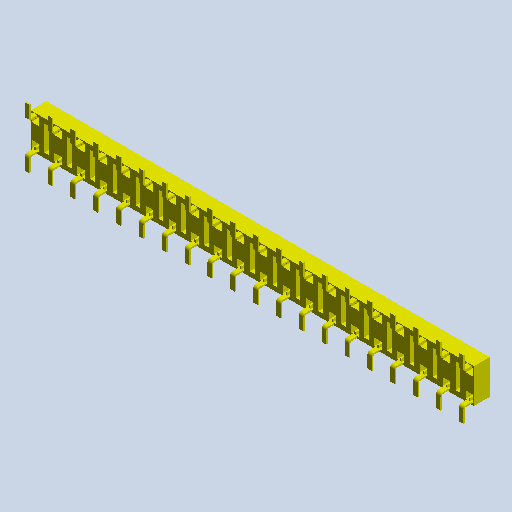
# Autodesk Inventor part: C-132-12-20-DV
Saved by Autodesk Inventor 2022 (Build 260153000, 153)
## iProperties
Category: PARTsolutions
Company: SAMTEC
Part Number: C-132-12-20-DV
Material: Generic
Catalog Web Link: www.cadenas.de
Description: C-132-Pins
Vendor: SAMTEC
Document SubType Name: Modeling
Designer: partserver
Manufacturer: SAMTEC
Mass: 0.2484 g
Surface Area: 10.7462 cm^2
Volume: 0.2484 cm^3
Density: 1 g/cm^3
Appearance: PSOLRGB-255-255-0
PSOL_IDENT_0: {$CADENAS_DATA\23d-libs\samtec\modelling\hle\parts\hle_pins.prj},176 {VTYP=3D},{NB=C-132-12-20-DV},{
PSOL_IDENT_1: LINA=C-132-12-20-DV},{NN=C-132},{DATE=08.04.2016 05:41:50},{GEOMDATE=08.04.2016 05:31:00},{VERSION=}
PSOL_IDENT_2: ,{LINEID=10},{WBVAR=POS,ESOPT},{WBNUMERIC=}  {NB=C-132-12-20-DV},{LINA=C-132-12-20-DV},{KT=DUMMY},{P
PSOL_IDENT_3: N=C-132-12-20-DV},{SERIES=HLE},{POSALG=  '02' , '-02' , '03' , '-03' , '04' , '-04' , '05' , '-05' ,
PSOL_IDENT_4: '06' , '-06' , '07' , '-07' , '08' , '-08' , '09' , '-09' , '10' , '-10' , '11' , '-11' , '12' , '-
PSOL_IDENT_5: 12' , '13' , '-13' , '14' , '-14' , '15' , '-15' , '16' , '-16' , '17' , '-17' , '18' , '-18' , '19'
PSOL_IDENT_6: , '-19' , '20' , '-20' , '21' , '-21' , '22' , '-22' , '23' , '-23' , '24' , '-24' , '25' , '-25' ,
PSOL_IDENT_7: '26' , '-26' , '27' , '-27' , '28' , '-28' , '29' , '-29' , '30' , '-30' , '31' , '-31' , '32' , '-
PSOL_IDENT_8: 32' , '33' , '-33' , '34' , '-34' , '35' , '-35' , '36' , '-36' , '37' , '-37' , '38' , '-38' , '39'
PSOL_IDENT_9: , '-39' , '40' , '-40'  , '41' , '-41' , '42' , '-42' , '43' , '-43' , '44' , '-44' , '45' , '-45'
PSOL_IDENT_10: , '46' , '-46' , '47' , '-47' , '48' , '-48' , '49' , '-49' , '50' , '-50'   , '51' , '-51' , '52' ,
PSOL_IDENT_11: '-52' , '53' , '-53' , '54' , '-54' , '55' , '-55' , '56' , '-56' , '57' , '-57' , '58' , '-58' , '
PSOL_IDENT_12: 59' , '-59' , '60' , '-60'  , '61' , '-61' , '62' , '-62' , '63' , '-63' , '64' , '-64' , '65' , '-6
PSOL_IDENT_13: 5' , '66' , '-66' , '67' , '-67' , '68' , '-68' , '69' , '-69' , '70' , '-70'  , '71' , '-71' , '72'
PSOL_IDENT_14: , '-72' , '73' , '-73' , '74' , '-74' , '75' , '-75'   },{POS=20},{LSALG=  '02' , '-02 - Surface Mo
PSOL_IDENT_15: unt'  },{LS=02},{ROPTALG=   'DV' , '-DV - Double Vertical'   },{ROPT=DV},{ESOPT=},{A=0.144},{B=0.138
PSOL_IDENT_16: },{L=2.000},{PINS=20},{H2=0.030},{W=0.2000},{PINH=0.025},{PINL=0.2590},{PINW=0.020},{PITCH=0.1000},{
PSOL_IDENT_17: PITCH2=0.1000},{X=0.045},{ESOPTPN=}
NB: C-132-12-20-DV
NN: C-132
NT: Pins
NBSYN: $PN.
LINA: C-132-12-20-DV
CATALOG: Samtec
PN: C-132-12-20-DV
SERIES: HLE
POS: -20
LS: 02
ROPT: DV
ESOPT: Standard
A: 0.144
B: 0.138
L: 2
H2: 0.03
W: 0.2
PINH: 0.025
PINL: 0.259
PINW: 0.02
PITCH: 0.1
PITCH2: 0.1
X: 0.045
SUPPLIER: SAMTEC
ARTICLENO: C-132-12-20-DV
BOMINFO: C-132-12-20-DV
CREATOR: CADENAS GmbH
Title: C-132-12-20-DV
Author: Cadenas PARTsolutions
Comments: Pins
Autodesk Inventor part; units mm, degrees
sketch "Sketch_11" plane through (0, 2.5146, 0) normal (0, 1, 0) x (1, 0, 0)
  line L0 (-24.638, 1.9177) -> (-24.638, -1.9177)
  line L1 (-24.638, -1.9177) -> (24.638, -1.9177)
  line L2 (24.638, -1.9177) -> (24.638, 1.9177)
  line L3 (24.638, 1.9177) -> (-24.638, 1.9177)
  line L4 (23.7236, -0.8636) -> (23.7236, -1.6764)
  line L5 (23.7236, -1.6764) -> (24.0538, -1.6764)
  line L6 (24.0538, -1.6764) -> (24.0538, -1.3716)
  line L7 (24.0538, -1.3716) -> (24.2062, -1.3716)
  line L8 (24.2062, -1.3716) -> (24.2062, -1.6764)
  line L9 (24.2062, -1.6764) -> (24.5364, -1.6764)
  line L10 (24.5364, -1.6764) -> (24.5364, -0.8636)
  line L11 (24.5364, -0.8636) -> (23.7236, -0.8636)
  line L12 (23.7236, 0.8636) -> (24.5364, 0.8636)
  line L13 (24.5364, 0.8636) -> (24.5364, 1.6764)
  line L14 (24.5364, 1.6764) -> (24.2062, 1.6764)
  line L15 (24.2062, 1.6764) -> (24.2062, 1.3716)
  line L16 (24.2062, 1.3716) -> (24.0538, 1.3716)
  line L17 (24.0538, 1.3716) -> (24.0538, 1.6764)
  line L18 (24.0538, 1.6764) -> (23.7236, 1.6764)
  line L19 (23.7236, 1.6764) -> (23.7236, 0.8636)
  line L20 (22.606, 1.397) -> (22.606, -1.397)
  line L21 (22.606, -1.397) -> (23.114, -1.397)
  line L22 (23.114, -1.397) -> (23.114, 1.397)
  line L23 (23.114, 1.397) -> (22.606, 1.397)
  line L24 (21.1836, -0.8636) -> (21.1836, -1.6764)
  line L25 (21.1836, -1.6764) -> (21.5138, -1.6764)
  line L26 (21.5138, -1.6764) -> (21.5138, -1.3716)
  line L27 (21.5138, -1.3716) -> (21.6662, -1.3716)
  line L28 (21.6662, -1.3716) -> (21.6662, -1.6764)
  line L29 (21.6662, -1.6764) -> (21.9964, -1.6764)
  line L30 (21.9964, -1.6764) -> (21.9964, -0.8636)
  line L31 (21.9964, -0.8636) -> (21.1836, -0.8636)
  line L32 (21.1836, 0.8636) -> (21.9964, 0.8636)
  line L33 (21.9964, 0.8636) -> (21.9964, 1.6764)
  line L34 (21.9964, 1.6764) -> (21.6662, 1.6764)
  line L35 (21.6662, 1.6764) -> (21.6662, 1.3716)
  line L36 (21.6662, 1.3716) -> (21.5138, 1.3716)
  line L37 (21.5138, 1.3716) -> (21.5138, 1.6764)
  line L38 (21.5138, 1.6764) -> (21.1836, 1.6764)
  line L39 (21.1836, 1.6764) -> (21.1836, 0.8636)
  line L40 (20.066, 1.397) -> (20.066, -1.397)
  line L41 (20.066, -1.397) -> (20.574, -1.397)
  line L42 (20.574, -1.397) -> (20.574, 1.397)
  line L43 (20.574, 1.397) -> (20.066, 1.397)
  line L44 (18.6436, -0.8636) -> (18.6436, -1.6764)
  line L45 (18.6436, -1.6764) -> (18.9738, -1.6764)
  line L46 (18.9738, -1.6764) -> (18.9738, -1.3716)
  line L47 (18.9738, -1.3716) -> (19.1262, -1.3716)
  line L48 (19.1262, -1.3716) -> (19.1262, -1.6764)
  line L49 (19.1262, -1.6764) -> (19.4564, -1.6764)
  line L50 (19.4564, -1.6764) -> (19.4564, -0.8636)
  line L51 (19.4564, -0.8636) -> (18.6436, -0.8636)
  line L52 (18.6436, 0.8636) -> (19.4564, 0.8636)
  line L53 (19.4564, 0.8636) -> (19.4564, 1.6764)
  line L54 (19.4564, 1.6764) -> (19.1262, 1.6764)
  line L55 (19.1262, 1.6764) -> (19.1262, 1.3716)
  line L56 (19.1262, 1.3716) -> (18.9738, 1.3716)
  line L57 (18.9738, 1.3716) -> (18.9738, 1.6764)
  line L58 (18.9738, 1.6764) -> (18.6436, 1.6764)
  line L59 (18.6436, 1.6764) -> (18.6436, 0.8636)
  line L60 (17.526, 1.397) -> (17.526, -1.397)
  line L61 (17.526, -1.397) -> (18.034, -1.397)
  line L62 (18.034, -1.397) -> (18.034, 1.397)
  line L63 (18.034, 1.397) -> (17.526, 1.397)
  line L64 (16.1036, -0.8636) -> (16.1036, -1.6764)
  line L65 (16.1036, -1.6764) -> (16.4338, -1.6764)
  line L66 (16.4338, -1.6764) -> (16.4338, -1.3716)
  line L67 (16.4338, -1.3716) -> (16.5862, -1.3716)
  line L68 (16.5862, -1.3716) -> (16.5862, -1.6764)
  line L69 (16.5862, -1.6764) -> (16.9164, -1.6764)
  line L70 (16.9164, -1.6764) -> (16.9164, -0.8636)
  line L71 (16.9164, -0.8636) -> (16.1036, -0.8636)
  line L72 (16.1036, 0.8636) -> (16.9164, 0.8636)
  line L73 (16.9164, 0.8636) -> (16.9164, 1.6764)
  line L74 (16.9164, 1.6764) -> (16.5862, 1.6764)
  line L75 (16.5862, 1.6764) -> (16.5862, 1.3716)
  line L76 (16.5862, 1.3716) -> (16.4338, 1.3716)
  line L77 (16.4338, 1.3716) -> (16.4338, 1.6764)
  line L78 (16.4338, 1.6764) -> (16.1036, 1.6764)
  line L79 (16.1036, 1.6764) -> (16.1036, 0.8636)
  line L80 (14.986, 1.397) -> (14.986, -1.397)
  line L81 (14.986, -1.397) -> (15.494, -1.397)
  line L82 (15.494, -1.397) -> (15.494, 1.397)
  line L83 (15.494, 1.397) -> (14.986, 1.397)
  line L84 (13.5636, -0.8636) -> (13.5636, -1.6764)
  line L85 (13.5636, -1.6764) -> (13.8938, -1.6764)
  line L86 (13.8938, -1.6764) -> (13.8938, -1.3716)
  line L87 (13.8938, -1.3716) -> (14.0462, -1.3716)
  line L88 (14.0462, -1.3716) -> (14.0462, -1.6764)
  line L89 (14.0462, -1.6764) -> (14.3764, -1.6764)
  line L90 (14.3764, -1.6764) -> (14.3764, -0.8636)
  line L91 (14.3764, -0.8636) -> (13.5636, -0.8636)
  line L92 (13.5636, 0.8636) -> (14.3764, 0.8636)
  line L93 (14.3764, 0.8636) -> (14.3764, 1.6764)
  line L94 (14.3764, 1.6764) -> (14.0462, 1.6764)
  line L95 (14.0462, 1.6764) -> (14.0462, 1.3716)
  line L96 (14.0462, 1.3716) -> (13.8938, 1.3716)
  line L97 (13.8938, 1.3716) -> (13.8938, 1.6764)
  line L98 (13.8938, 1.6764) -> (13.5636, 1.6764)
  line L99 (13.5636, 1.6764) -> (13.5636, 0.8636)
  line L100 (12.446, 1.397) -> (12.446, -1.397)
  line L101 (12.446, -1.397) -> (12.954, -1.397)
  line L102 (12.954, -1.397) -> (12.954, 1.397)
  line L103 (12.954, 1.397) -> (12.446, 1.397)
  line L104 (11.0236, -0.8636) -> (11.0236, -1.6764)
  line L105 (11.0236, -1.6764) -> (11.3538, -1.6764)
  line L106 (11.3538, -1.6764) -> (11.3538, -1.3716)
  line L107 (11.3538, -1.3716) -> (11.5062, -1.3716)
  line L108 (11.5062, -1.3716) -> (11.5062, -1.6764)
  line L109 (11.5062, -1.6764) -> (11.8364, -1.6764)
  line L110 (11.8364, -1.6764) -> (11.8364, -0.8636)
  line L111 (11.8364, -0.8636) -> (11.0236, -0.8636)
  line L112 (11.0236, 0.8636) -> (11.8364, 0.8636)
  line L113 (11.8364, 0.8636) -> (11.8364, 1.6764)
  line L114 (11.8364, 1.6764) -> (11.5062, 1.6764)
  line L115 (11.5062, 1.6764) -> (11.5062, 1.3716)
  line L116 (11.5062, 1.3716) -> (11.3538, 1.3716)
  line L117 (11.3538, 1.3716) -> (11.3538, 1.6764)
  line L118 (11.3538, 1.6764) -> (11.0236, 1.6764)
  line L119 (11.0236, 1.6764) -> (11.0236, 0.8636)
  line L120 (9.906, 1.397) -> (9.906, -1.397)
  line L121 (9.906, -1.397) -> (10.414, -1.397)
  line L122 (10.414, -1.397) -> (10.414, 1.397)
  line L123 (10.414, 1.397) -> (9.906, 1.397)
  line L124 (8.4836, -0.8636) -> (8.4836, -1.6764)
  line L125 (8.4836, -1.6764) -> (8.8138, -1.6764)
  line L126 (8.8138, -1.6764) -> (8.8138, -1.3716)
  line L127 (8.8138, -1.3716) -> (8.9662, -1.3716)
  line L128 (8.9662, -1.3716) -> (8.9662, -1.6764)
  line L129 (8.9662, -1.6764) -> (9.2964, -1.6764)
  line L130 (9.2964, -1.6764) -> (9.2964, -0.8636)
  line L131 (9.2964, -0.8636) -> (8.4836, -0.8636)
  line L132 (8.4836, 0.8636) -> (9.2964, 0.8636)
  line L133 (9.2964, 0.8636) -> (9.2964, 1.6764)
  line L134 (9.2964, 1.6764) -> (8.9662, 1.6764)
  line L135 (8.9662, 1.6764) -> (8.9662, 1.3716)
  line L136 (8.9662, 1.3716) -> (8.8138, 1.3716)
  line L137 (8.8138, 1.3716) -> (8.8138, 1.6764)
  line L138 (8.8138, 1.6764) -> (8.4836, 1.6764)
  line L139 (8.4836, 1.6764) -> (8.4836, 0.8636)
  line L140 (7.366, 1.397) -> (7.366, -1.397)
  line L141 (7.366, -1.397) -> (7.874, -1.397)
  line L142 (7.874, -1.397) -> (7.874, 1.397)
  line L143 (7.874, 1.397) -> (7.366, 1.397)
  line L144 (5.9436, -0.8636) -> (5.9436, -1.6764)
  line L145 (5.9436, -1.6764) -> (6.2738, -1.6764)
  line L146 (6.2738, -1.6764) -> (6.2738, -1.3716)
  line L147 (6.2738, -1.3716) -> (6.4262, -1.3716)
  line L148 (6.4262, -1.3716) -> (6.4262, -1.6764)
  line L149 (6.4262, -1.6764) -> (6.7564, -1.6764)
  line L150 (6.7564, -1.6764) -> (6.7564, -0.8636)
  line L151 (6.7564, -0.8636) -> (5.9436, -0.8636)
  line L152 (5.9436, 0.8636) -> (6.7564, 0.8636)
  line L153 (6.7564, 0.8636) -> (6.7564, 1.6764)
  line L154 (6.7564, 1.6764) -> (6.4262, 1.6764)
  line L155 (6.4262, 1.6764) -> (6.4262, 1.3716)
  line L156 (6.4262, 1.3716) -> (6.2738, 1.3716)
  line L157 (6.2738, 1.3716) -> (6.2738, 1.6764)
  line L158 (6.2738, 1.6764) -> (5.9436, 1.6764)
  line L159 (5.9436, 1.6764) -> (5.9436, 0.8636)
  line L160 (4.826, 1.397) -> (4.826, -1.397)
  line L161 (4.826, -1.397) -> (5.334, -1.397)
  line L162 (5.334, -1.397) -> (5.334, 1.397)
  line L163 (5.334, 1.397) -> (4.826, 1.397)
  line L164 (3.4036, -0.8636) -> (3.4036, -1.6764)
  line L165 (3.4036, -1.6764) -> (3.7338, -1.6764)
  line L166 (3.7338, -1.6764) -> (3.7338, -1.3716)
  line L167 (3.7338, -1.3716) -> (3.8862, -1.3716)
  line L168 (3.8862, -1.3716) -> (3.8862, -1.6764)
  line L169 (3.8862, -1.6764) -> (4.2164, -1.6764)
  line L170 (4.2164, -1.6764) -> (4.2164, -0.8636)
  line L171 (4.2164, -0.8636) -> (3.4036, -0.8636)
  line L172 (3.4036, 0.8636) -> (4.2164, 0.8636)
  line L173 (4.2164, 0.8636) -> (4.2164, 1.6764)
  line L174 (4.2164, 1.6764) -> (3.8862, 1.6764)
  line L175 (3.8862, 1.6764) -> (3.8862, 1.3716)
  line L176 (3.8862, 1.3716) -> (3.7338, 1.3716)
  line L177 (3.7338, 1.3716) -> (3.7338, 1.6764)
  line L178 (3.7338, 1.6764) -> (3.4036, 1.6764)
  line L179 (3.4036, 1.6764) -> (3.4036, 0.8636)
  line L180 (2.286, 1.397) -> (2.286, -1.397)
  line L181 (2.286, -1.397) -> (2.794, -1.397)
  line L182 (2.794, -1.397) -> (2.794, 1.397)
  line L183 (2.794, 1.397) -> (2.286, 1.397)
  line L184 (0.8636, -0.8636) -> (0.8636, -1.6764)
  line L185 (0.8636, -1.6764) -> (1.1938, -1.6764)
  line L186 (1.1938, -1.6764) -> (1.1938, -1.3716)
  line L187 (1.1938, -1.3716) -> (1.3462, -1.3716)
  line L188 (1.3462, -1.3716) -> (1.3462, -1.6764)
  line L189 (1.3462, -1.6764) -> (1.6764, -1.6764)
  line L190 (1.6764, -1.6764) -> (1.6764, -0.8636)
  line L191 (1.6764, -0.8636) -> (0.8636, -0.8636)
  line L192 (0.8636, 0.8636) -> (1.6764, 0.8636)
  line L193 (1.6764, 0.8636) -> (1.6764, 1.6764)
  line L194 (1.6764, 1.6764) -> (1.3462, 1.6764)
  line L195 (1.3462, 1.6764) -> (1.3462, 1.3716)
  line L196 (1.3462, 1.3716) -> (1.1938, 1.3716)
  line L197 (1.1938, 1.3716) -> (1.1938, 1.6764)
  line L198 (1.1938, 1.6764) -> (0.8636, 1.6764)
  line L199 (0.8636, 1.6764) -> (0.8636, 0.8636)
  line L200 (-0.254, 1.397) -> (-0.254, -1.397)
  line L201 (-0.254, -1.397) -> (0.254, -1.397)
  line L202 (0.254, -1.397) -> (0.254, 1.397)
  line L203 (0.254, 1.397) -> (-0.254, 1.397)
  line L204 (-1.6764, -0.8636) -> (-1.6764, -1.6764)
  line L205 (-1.6764, -1.6764) -> (-1.3462, -1.6764)
  line L206 (-1.3462, -1.6764) -> (-1.3462, -1.3716)
  line L207 (-1.3462, -1.3716) -> (-1.1938, -1.3716)
  line L208 (-1.1938, -1.3716) -> (-1.1938, -1.6764)
  line L209 (-1.1938, -1.6764) -> (-0.8636, -1.6764)
  line L210 (-0.8636, -1.6764) -> (-0.8636, -0.8636)
  line L211 (-0.8636, -0.8636) -> (-1.6764, -0.8636)
  line L212 (-1.6764, 0.8636) -> (-0.8636, 0.8636)
  line L213 (-0.8636, 0.8636) -> (-0.8636, 1.6764)
  line L214 (-0.8636, 1.6764) -> (-1.1938, 1.6764)
  line L215 (-1.1938, 1.6764) -> (-1.1938, 1.3716)
  line L216 (-1.1938, 1.3716) -> (-1.3462, 1.3716)
  line L217 (-1.3462, 1.3716) -> (-1.3462, 1.6764)
  line L218 (-1.3462, 1.6764) -> (-1.6764, 1.6764)
  line L219 (-1.6764, 1.6764) -> (-1.6764, 0.8636)
  line L220 (-2.794, 1.397) -> (-2.794, -1.397)
  line L221 (-2.794, -1.397) -> (-2.286, -1.397)
  line L222 (-2.286, -1.397) -> (-2.286, 1.397)
  line L223 (-2.286, 1.397) -> (-2.794, 1.397)
  line L224 (-4.2164, -0.8636) -> (-4.2164, -1.6764)
  line L225 (-4.2164, -1.6764) -> (-3.8862, -1.6764)
  line L226 (-3.8862, -1.6764) -> (-3.8862, -1.3716)
  line L227 (-3.8862, -1.3716) -> (-3.7338, -1.3716)
  line L228 (-3.7338, -1.3716) -> (-3.7338, -1.6764)
  line L229 (-3.7338, -1.6764) -> (-3.4036, -1.6764)
  line L230 (-3.4036, -1.6764) -> (-3.4036, -0.8636)
  line L231 (-3.4036, -0.8636) -> (-4.2164, -0.8636)
  line L232 (-4.2164, 0.8636) -> (-3.4036, 0.8636)
  line L233 (-3.4036, 0.8636) -> (-3.4036, 1.6764)
  line L234 (-3.4036, 1.6764) -> (-3.7338, 1.6764)
  line L235 (-3.7338, 1.6764) -> (-3.7338, 1.3716)
  line L236 (-3.7338, 1.3716) -> (-3.8862, 1.3716)
  line L237 (-3.8862, 1.3716) -> (-3.8862, 1.6764)
  line L238 (-3.8862, 1.6764) -> (-4.2164, 1.6764)
  line L239 (-4.2164, 1.6764) -> (-4.2164, 0.8636)
  line L240 (-5.334, 1.397) -> (-5.334, -1.397)
  line L241 (-5.334, -1.397) -> (-4.826, -1.397)
  line L242 (-4.826, -1.397) -> (-4.826, 1.397)
  line L243 (-4.826, 1.397) -> (-5.334, 1.397)
  line L244 (-6.7564, -0.8636) -> (-6.7564, -1.6764)
  line L245 (-6.7564, -1.6764) -> (-6.4262, -1.6764)
  line L246 (-6.4262, -1.6764) -> (-6.4262, -1.3716)
  line L247 (-6.4262, -1.3716) -> (-6.2738, -1.3716)
  line L248 (-6.2738, -1.3716) -> (-6.2738, -1.6764)
  line L249 (-6.2738, -1.6764) -> (-5.9436, -1.6764)
  line L250 (-5.9436, -1.6764) -> (-5.9436, -0.8636)
  line L251 (-5.9436, -0.8636) -> (-6.7564, -0.8636)
  line L252 (-6.7564, 0.8636) -> (-5.9436, 0.8636)
  line L253 (-5.9436, 0.8636) -> (-5.9436, 1.6764)
  line L254 (-5.9436, 1.6764) -> (-6.2738, 1.6764)
  line L255 (-6.2738, 1.6764) -> (-6.2738, 1.3716)
  line L256 (-6.2738, 1.3716) -> (-6.4262, 1.3716)
  line L257 (-6.4262, 1.3716) -> (-6.4262, 1.6764)
  line L258 (-6.4262, 1.6764) -> (-6.7564, 1.6764)
  line L259 (-6.7564, 1.6764) -> (-6.7564, 0.8636)
  line L260 (-7.874, 1.397) -> (-7.874, -1.397)
  line L261 (-7.874, -1.397) -> (-7.366, -1.397)
  line L262 (-7.366, -1.397) -> (-7.366, 1.397)
  line L263 (-7.366, 1.397) -> (-7.874, 1.397)
  line L264 (-9.2964, -0.8636) -> (-9.2964, -1.6764)
  line L265 (-9.2964, -1.6764) -> (-8.9662, -1.6764)
  line L266 (-8.9662, -1.6764) -> (-8.9662, -1.3716)
  line L267 (-8.9662, -1.3716) -> (-8.8138, -1.3716)
  line L268 (-8.8138, -1.3716) -> (-8.8138, -1.6764)
  line L269 (-8.8138, -1.6764) -> (-8.4836, -1.6764)
  line L270 (-8.4836, -1.6764) -> (-8.4836, -0.8636)
  line L271 (-8.4836, -0.8636) -> (-9.2964, -0.8636)
  line L272 (-9.2964, 0.8636) -> (-8.4836, 0.8636)
  line L273 (-8.4836, 0.8636) -> (-8.4836, 1.6764)
  line L274 (-8.4836, 1.6764) -> (-8.8138, 1.6764)
  line L275 (-8.8138, 1.6764) -> (-8.8138, 1.3716)
  line L276 (-8.8138, 1.3716) -> (-8.9662, 1.3716)
  line L277 (-8.9662, 1.3716) -> (-8.9662, 1.6764)
  line L278 (-8.9662, 1.6764) -> (-9.2964, 1.6764)
  line L279 (-9.2964, 1.6764) -> (-9.2964, 0.8636)
  line L280 (-10.414, 1.397) -> (-10.414, -1.397)
  line L281 (-10.414, -1.397) -> (-9.906, -1.397)
  line L282 (-9.906, -1.397) -> (-9.906, 1.397)
  line L283 (-9.906, 1.397) -> (-10.414, 1.397)
  line L284 (-11.8364, -0.8636) -> (-11.8364, -1.6764)
  line L285 (-11.8364, -1.6764) -> (-11.5062, -1.6764)
  line L286 (-11.5062, -1.6764) -> (-11.5062, -1.3716)
  line L287 (-11.5062, -1.3716) -> (-11.3538, -1.3716)
  line L288 (-11.3538, -1.3716) -> (-11.3538, -1.6764)
  line L289 (-11.3538, -1.6764) -> (-11.0236, -1.6764)
  line L290 (-11.0236, -1.6764) -> (-11.0236, -0.8636)
  line L291 (-11.0236, -0.8636) -> (-11.8364, -0.8636)
  line L292 (-11.8364, 0.8636) -> (-11.0236, 0.8636)
  line L293 (-11.0236, 0.8636) -> (-11.0236, 1.6764)
  line L294 (-11.0236, 1.6764) -> (-11.3538, 1.6764)
  line L295 (-11.3538, 1.6764) -> (-11.3538, 1.3716)
  line L296 (-11.3538, 1.3716) -> (-11.5062, 1.3716)
  line L297 (-11.5062, 1.3716) -> (-11.5062, 1.6764)
  line L298 (-11.5062, 1.6764) -> (-11.8364, 1.6764)
  line L299 (-11.8364, 1.6764) -> (-11.8364, 0.8636)
  line L300 (-12.954, 1.397) -> (-12.954, -1.397)
  line L301 (-12.954, -1.397) -> (-12.446, -1.397)
  line L302 (-12.446, -1.397) -> (-12.446, 1.397)
  line L303 (-12.446, 1.397) -> (-12.954, 1.397)
  line L304 (-14.3764, -0.8636) -> (-14.3764, -1.6764)
  line L305 (-14.3764, -1.6764) -> (-14.0462, -1.6764)
  line L306 (-14.0462, -1.6764) -> (-14.0462, -1.3716)
  line L307 (-14.0462, -1.3716) -> (-13.8938, -1.3716)
  line L308 (-13.8938, -1.3716) -> (-13.8938, -1.6764)
  line L309 (-13.8938, -1.6764) -> (-13.5636, -1.6764)
  line L310 (-13.5636, -1.6764) -> (-13.5636, -0.8636)
  line L311 (-13.5636, -0.8636) -> (-14.3764, -0.8636)
  line L312 (-14.3764, 0.8636) -> (-13.5636, 0.8636)
  line L313 (-13.5636, 0.8636) -> (-13.5636, 1.6764)
  line L314 (-13.5636, 1.6764) -> (-13.8938, 1.6764)
  line L315 (-13.8938, 1.6764) -> (-13.8938, 1.3716)
  line L316 (-13.8938, 1.3716) -> (-14.0462, 1.3716)
  line L317 (-14.0462, 1.3716) -> (-14.0462, 1.6764)
  line L318 (-14.0462, 1.6764) -> (-14.3764, 1.6764)
  line L319 (-14.3764, 1.6764) -> (-14.3764, 0.8636)
  line L320 (-15.494, 1.397) -> (-15.494, -1.397)
  line L321 (-15.494, -1.397) -> (-14.986, -1.397)
  line L322 (-14.986, -1.397) -> (-14.986, 1.397)
  line L323 (-14.986, 1.397) -> (-15.494, 1.397)
  line L324 (-16.9164, -0.8636) -> (-16.9164, -1.6764)
  line L325 (-16.9164, -1.6764) -> (-16.5862, -1.6764)
  line L326 (-16.5862, -1.6764) -> (-16.5862, -1.3716)
  line L327 (-16.5862, -1.3716) -> (-16.4338, -1.3716)
  line L328 (-16.4338, -1.3716) -> (-16.4338, -1.6764)
  line L329 (-16.4338, -1.6764) -> (-16.1036, -1.6764)
  line L330 (-16.1036, -1.6764) -> (-16.1036, -0.8636)
  line L331 (-16.1036, -0.8636) -> (-16.9164, -0.8636)
  line L332 (-16.9164, 0.8636) -> (-16.1036, 0.8636)
  line L333 (-16.1036, 0.8636) -> (-16.1036, 1.6764)
  line L334 (-16.1036, 1.6764) -> (-16.4338, 1.6764)
  line L335 (-16.4338, 1.6764) -> (-16.4338, 1.3716)
  line L336 (-16.4338, 1.3716) -> (-16.5862, 1.3716)
  line L337 (-16.5862, 1.3716) -> (-16.5862, 1.6764)
  line L338 (-16.5862, 1.6764) -> (-16.9164, 1.6764)
  line L339 (-16.9164, 1.6764) -> (-16.9164, 0.8636)
  line L340 (-18.034, 1.397) -> (-18.034, -1.397)
  line L341 (-18.034, -1.397) -> (-17.526, -1.397)
  line L342 (-17.526, -1.397) -> (-17.526, 1.397)
  line L343 (-17.526, 1.397) -> (-18.034, 1.397)
  line L344 (-19.4564, -0.8636) -> (-19.4564, -1.6764)
  line L345 (-19.4564, -1.6764) -> (-19.1262, -1.6764)
  line L346 (-19.1262, -1.6764) -> (-19.1262, -1.3716)
  line L347 (-19.1262, -1.3716) -> (-18.9738, -1.3716)
  line L348 (-18.9738, -1.3716) -> (-18.9738, -1.6764)
  line L349 (-18.9738, -1.6764) -> (-18.6436, -1.6764)
  line L350 (-18.6436, -1.6764) -> (-18.6436, -0.8636)
  line L351 (-18.6436, -0.8636) -> (-19.4564, -0.8636)
  line L352 (-19.4564, 0.8636) -> (-18.6436, 0.8636)
  line L353 (-18.6436, 0.8636) -> (-18.6436, 1.6764)
  line L354 (-18.6436, 1.6764) -> (-18.9738, 1.6764)
  line L355 (-18.9738, 1.6764) -> (-18.9738, 1.3716)
  line L356 (-18.9738, 1.3716) -> (-19.1262, 1.3716)
  line L357 (-19.1262, 1.3716) -> (-19.1262, 1.6764)
  line L358 (-19.1262, 1.6764) -> (-19.4564, 1.6764)
  line L359 (-19.4564, 1.6764) -> (-19.4564, 0.8636)
  line L360 (-20.574, 1.397) -> (-20.574, -1.397)
  line L361 (-20.574, -1.397) -> (-20.066, -1.397)
  line L362 (-20.066, -1.397) -> (-20.066, 1.397)
  line L363 (-20.066, 1.397) -> (-20.574, 1.397)
  line L364 (-21.9964, -0.8636) -> (-21.9964, -1.6764)
  line L365 (-21.9964, -1.6764) -> (-21.6662, -1.6764)
  line L366 (-21.6662, -1.6764) -> (-21.6662, -1.3716)
  line L367 (-21.6662, -1.3716) -> (-21.5138, -1.3716)
  line L368 (-21.5138, -1.3716) -> (-21.5138, -1.6764)
  line L369 (-21.5138, -1.6764) -> (-21.1836, -1.6764)
  line L370 (-21.1836, -1.6764) -> (-21.1836, -0.8636)
  line L371 (-21.1836, -0.8636) -> (-21.9964, -0.8636)
  line L372 (-21.9964, 0.8636) -> (-21.1836, 0.8636)
  line L373 (-21.1836, 0.8636) -> (-21.1836, 1.6764)
  line L374 (-21.1836, 1.6764) -> (-21.5138, 1.6764)
  line L375 (-21.5138, 1.6764) -> (-21.5138, 1.3716)
  line L376 (-21.5138, 1.3716) -> (-21.6662, 1.3716)
  line L377 (-21.6662, 1.3716) -> (-21.6662, 1.6764)
  line L378 (-21.6662, 1.6764) -> (-21.9964, 1.6764)
  line L379 (-21.9964, 1.6764) -> (-21.9964, 0.8636)
  line L380 (-23.114, 1.397) -> (-23.114, -1.397)
  line L381 (-23.114, -1.397) -> (-22.606, -1.397)
  line L382 (-22.606, -1.397) -> (-22.606, 1.397)
  line L383 (-22.606, 1.397) -> (-23.114, 1.397)
  line L384 (-24.5364, -0.8636) -> (-24.5364, -1.6764)
  line L385 (-24.5364, -1.6764) -> (-24.2062, -1.6764)
  line L386 (-24.2062, -1.6764) -> (-24.2062, -1.3716)
  line L387 (-24.2062, -1.3716) -> (-24.0538, -1.3716)
  line L388 (-24.0538, -1.3716) -> (-24.0538, -1.6764)
  line L389 (-24.0538, -1.6764) -> (-23.7236, -1.6764)
  line L390 (-23.7236, -1.6764) -> (-23.7236, -0.8636)
  line L391 (-23.7236, -0.8636) -> (-24.5364, -0.8636)
  line L392 (-24.5364, 0.8636) -> (-23.7236, 0.8636)
  line L393 (-23.7236, 0.8636) -> (-23.7236, 1.6764)
  line L394 (-23.7236, 1.6764) -> (-24.0538, 1.6764)
  line L395 (-24.0538, 1.6764) -> (-24.0538, 1.3716)
  line L396 (-24.0538, 1.3716) -> (-24.2062, 1.3716)
  line L397 (-24.2062, 1.3716) -> (-24.2062, 1.6764)
  line L398 (-24.2062, 1.6764) -> (-24.5364, 1.6764)
  line L399 (-24.5364, 1.6764) -> (-24.5364, 0.8636)
  constraints: 800 end point
extrude "Extrusion1" add sketch "Sketch_11" against normal blind 1.7526
sketch "Sketch_12" plane through (0, 0, 0) normal (1, 0, 0) x (0, 1, 0)
  line L0 (-0.1524, 3.2893) -> (-0.1524, 1.9558)
  arc A0 (-0.1524, 1.9558) -> (0.1524, 1.651) centre (0.1524, 1.9558) ccw
  line L1 (0.1524, 1.651) -> (0.762, 1.651)
  line L2 (0.762, 1.651) -> (0.762, 1.8288)
  line L3 (0.762, 1.8288) -> (0.127, 1.8288)
  arc A1 (0, 1.9558) -> (0.127, 1.8288) centre (0.127, 1.9558) ccw
  line L4 (0, 1.9558) -> (0, 3.2893)
  line L5 (0, 3.2893) -> (-0.1524, 3.2893)
  constraints: 12 end point, 4 point on circle, 2 centre point
extrude "Extrusion2" add sketch "Sketch_12" along normal mid plane 49.276
sketch "Sketch_13" plane through (0, 0, 0) normal (1, 0, 0) x (0, 1, 0)
  arc A0 (0.1524, -1.651) -> (-0.1524, -1.9558) centre (0.1524, -1.9558) ccw
  line L0 (-0.1524, -1.9558) -> (-0.1524, -3.2893)
  line L1 (-0.1524, -3.2893) -> (0, -3.2893)
  line L2 (0, -3.2893) -> (0, -1.9558)
  arc A1 (0.127, -1.8288) -> (0, -1.9558) centre (0.127, -1.9558) ccw
  line L3 (0.127, -1.8288) -> (0.762, -1.8288)
  line L4 (0.762, -1.8288) -> (0.762, -1.651)
  line L5 (0.762, -1.651) -> (0.1524, -1.651)
  constraints: 12 end point, 4 point on circle, 2 centre point
extrude "Extrusion3" add sketch "Sketch_13" along normal mid plane 49.276
sketch "Sketch_5" plane through (0, 0, 0) normal (0, 0, 1) x (1, 0, 0)
  line L0 (-26.924, -3.556) -> (26.416, -3.556)
  line L1 (26.416, -3.556) -> (26.416, 0.762)
  line L2 (26.416, 0.762) -> (24.384, 0.762)
  line L3 (24.384, 0.762) -> (24.384, -3.048)
  line L4 (24.384, -3.048) -> (23.876, -3.048)
  line L5 (23.876, -3.048) -> (23.876, 0.762)
  line L6 (23.876, 0.762) -> (21.844, 0.762)
  line L7 (21.844, 0.762) -> (21.844, -3.048)
  line L8 (21.844, -3.048) -> (21.336, -3.048)
  line L9 (21.336, -3.048) -> (21.336, 0.762)
  line L10 (21.336, 0.762) -> (19.304, 0.762)
  line L11 (19.304, 0.762) -> (19.304, -3.048)
  line L12 (19.304, -3.048) -> (18.796, -3.048)
  line L13 (18.796, -3.048) -> (18.796, 0.762)
  line L14 (18.796, 0.762) -> (16.764, 0.762)
  line L15 (16.764, 0.762) -> (16.764, -3.048)
  line L16 (16.764, -3.048) -> (16.256, -3.048)
  line L17 (16.256, -3.048) -> (16.256, 0.762)
  line L18 (16.256, 0.762) -> (14.224, 0.762)
  line L19 (14.224, 0.762) -> (14.224, -3.048)
  line L20 (14.224, -3.048) -> (13.716, -3.048)
  line L21 (13.716, -3.048) -> (13.716, 0.762)
  line L22 (13.716, 0.762) -> (11.684, 0.762)
  line L23 (11.684, 0.762) -> (11.684, -3.048)
  line L24 (11.684, -3.048) -> (11.176, -3.048)
  line L25 (11.176, -3.048) -> (11.176, 0.762)
  line L26 (11.176, 0.762) -> (9.144, 0.762)
  line L27 (9.144, 0.762) -> (9.144, -3.048)
  line L28 (9.144, -3.048) -> (8.636, -3.048)
  line L29 (8.636, -3.048) -> (8.636, 0.762)
  line L30 (8.636, 0.762) -> (6.604, 0.762)
  line L31 (6.604, 0.762) -> (6.604, -3.048)
  line L32 (6.604, -3.048) -> (6.096, -3.048)
  line L33 (6.096, -3.048) -> (6.096, 0.762)
  line L34 (6.096, 0.762) -> (4.064, 0.762)
  line L35 (4.064, 0.762) -> (4.064, -3.048)
  line L36 (4.064, -3.048) -> (3.556, -3.048)
  line L37 (3.556, -3.048) -> (3.556, 0.762)
  line L38 (3.556, 0.762) -> (1.524, 0.762)
  line L39 (1.524, 0.762) -> (1.524, -3.048)
  line L40 (1.524, -3.048) -> (1.016, -3.048)
  line L41 (1.016, -3.048) -> (1.016, 0.762)
  line L42 (1.016, 0.762) -> (-1.016, 0.762)
  line L43 (-1.016, 0.762) -> (-1.016, -3.048)
  line L44 (-1.016, -3.048) -> (-1.524, -3.048)
  line L45 (-1.524, -3.048) -> (-1.524, 0.762)
  line L46 (-1.524, 0.762) -> (-3.556, 0.762)
  line L47 (-3.556, 0.762) -> (-3.556, -3.048)
  line L48 (-3.556, -3.048) -> (-4.064, -3.048)
  line L49 (-4.064, -3.048) -> (-4.064, 0.762)
  line L50 (-4.064, 0.762) -> (-6.096, 0.762)
  line L51 (-6.096, 0.762) -> (-6.096, -3.048)
  line L52 (-6.096, -3.048) -> (-6.604, -3.048)
  line L53 (-6.604, -3.048) -> (-6.604, 0.762)
  line L54 (-6.604, 0.762) -> (-8.636, 0.762)
  line L55 (-8.636, 0.762) -> (-8.636, -3.048)
  line L56 (-8.636, -3.048) -> (-9.144, -3.048)
  line L57 (-9.144, -3.048) -> (-9.144, 0.762)
  line L58 (-9.144, 0.762) -> (-11.176, 0.762)
  line L59 (-11.176, 0.762) -> (-11.176, -3.048)
  line L60 (-11.176, -3.048) -> (-11.684, -3.048)
  line L61 (-11.684, -3.048) -> (-11.684, 0.762)
  line L62 (-11.684, 0.762) -> (-13.716, 0.762)
  line L63 (-13.716, 0.762) -> (-13.716, -3.048)
  line L64 (-13.716, -3.048) -> (-14.224, -3.048)
  line L65 (-14.224, -3.048) -> (-14.224, 0.762)
  line L66 (-14.224, 0.762) -> (-16.256, 0.762)
  line L67 (-16.256, 0.762) -> (-16.256, -3.048)
  line L68 (-16.256, -3.048) -> (-16.764, -3.048)
  line L69 (-16.764, -3.048) -> (-16.764, 0.762)
  line L70 (-16.764, 0.762) -> (-18.796, 0.762)
  line L71 (-18.796, 0.762) -> (-18.796, -3.048)
  line L72 (-18.796, -3.048) -> (-19.304, -3.048)
  line L73 (-19.304, -3.048) -> (-19.304, 0.762)
  line L74 (-19.304, 0.762) -> (-21.336, 0.762)
  line L75 (-21.336, 0.762) -> (-21.336, -3.048)
  line L76 (-21.336, -3.048) -> (-21.844, -3.048)
  line L77 (-21.844, -3.048) -> (-21.844, 0.762)
  line L78 (-21.844, 0.762) -> (-23.876, 0.762)
  line L79 (-23.876, 0.762) -> (-23.876, -3.048)
  line L80 (-23.876, -3.048) -> (-24.384, -3.048)
  line L81 (-24.384, -3.048) -> (-24.384, 0.762)
  line L82 (-24.384, 0.762) -> (-26.924, 0.762)
  line L83 (-26.924, 0.762) -> (-26.924, -3.556)
  constraints: 168 end point
extrude "Extrusion4" cut sketch "Sketch_5" along normal mid plane 10.16
ref_plane "pins_to_socket_XY" through (0, 0, 0) normal (0, 1, 0) x (1, 0, 0)
ref_plane "pins_to_socket_YZ" through (0, 0, 0) normal (1, 0, 0) x (0, 0, -1)
ref_plane "pins_to_socket_ZX" through (0, 0, 0) normal (0, 0, -1) x (0, 1, 0)
body "Solid1"
